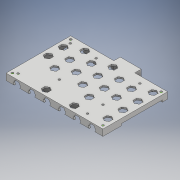
# Autodesk Inventor part: Housing Bottom
Saved by Autodesk Inventor 2017 (Build 210142000, 142)
## iProperties
Created: 2017-05-04
Part Number: Housing Bottom
Material: Generic
Document SubType Name: Modeling
Designer: andrew
Density: 1 g/cm^3
Appearance: Default
Author: andrew
Autodesk Inventor part; units mm, degrees
(part 1 of 3)
ref_plane "YZ Plane" through (0, 0, 0) normal (1, 0, 0) x (0, 1, 0)
ref_plane "XZ Plane" through (0, 0, 0) normal (0, 1, 0) x (-1, 0, 0)
ref_plane "XY Plane" through (0, 0, 0) normal (0, 0, 1) x (1, 0, 0)
sketch "Sketch1" plane through (0, 0, 0) normal (0, 0, 1) x (1, 0, 0)
  line L0 (0, 0) -> (122, 0) construction
  line L1 (122, 78) -> (0, 78) construction
  line L2 (0, 78) -> (0, 0) construction
  line L3 (122, 78) -> (124, 78) construction
  line L4 (124, 78) -> (124, 0) construction
  line L5 (124, 0) -> (122, 0) construction
  line L6 (122, 0) -> (122, 78) construction
  line L7 (0, 78) -> (124, 78) construction
  line L8 (124, 81) -> (0, 81) construction
  line L9 (0, 81) -> (0, 78) construction
  line L10 (124, 78) -> (124, 81) construction
  line L11 (124, 78) -> (124, 81) construction
  line L12 (0, 77.4184) -> (0, 81) construction
  line L13 (0, 81) -> (124, 81) construction
  line L14 (0, 81) -> (124, 81) construction
  line L15 (124, 0) -> (0, 0) construction
  line L16 (0, 0) -> (0, 81) construction
  line L17 (0, 81) -> (124, 81) construction
  line L18 (124, 81) -> (124, 0) construction
  line L19 (124, 0) -> (0, 0) construction
  line L20 (0, 0) -> (0, 81) construction
  line L21 (122, 78) -> (37, 78) construction
  line L22 (37, 78) -> (37, 22) construction
  line L23 (37, 22) -> (122, 22) construction
  line L24 (122, 22) -> (122, 78) construction
  line L25 (37, 22) -> (40.5, 22) construction
  line L26 (40.5, 22) -> (40.5, 25.5) construction
  line L27 (40.5, 25.5) -> (37, 25.5) construction
  line L28 (37, 25.5) -> (37, 22) construction
  line L29 (40.5, 25.5) -> (40.5, 74.5) construction
  circle A0 centre (40.5, 74.5) radius 1.375
  circle A1 centre (40.5, 25.5) radius 1.375
  circle A2 centre (98.5, 74.5) radius 1.375
  line L30 (0, 81) -> (124, 81) construction
  line L31 (124, 81) -> (124, 0) construction
  line L32 (124, 0) -> (0, 0) construction
  line L33 (0, 0) -> (0, 81) construction
  line L34 (124, 81.5) -> (0, 81.5) construction
  line L35 (122, -0.5) -> (-0.5, -0.5) construction
  line L36 (-0.5, -0.5) -> (-0.5, 78) construction
  line L37 (-0.5, 78) -> (-0.5, 81) construction
  line L38 (124, 81.5) -> (124.5, 81.5) construction
  line L39 (37, 78) -> (69, 78) construction
  line L40 (69, 78) -> (81, 78) construction
  line L41 (81, 78) -> (81, 90) construction
  line L42 (81, 90) -> (57, 90) construction
  line L43 (57, 90) -> (57, 78) construction
  line L44 (37, 78) -> (47.6, 78) construction
  line L45 (47.6, 78) -> (47.6, 82.811) construction
  line L46 (47.6, 82.811) -> (53.1, 82.811) construction
  line L47 (53.1, 82.811) -> (42.1, 82.811) construction
  line L48 (42.1, 82.811) -> (42.1, 78) construction
  line L49 (53.1, 82.811) -> (53.1, 78) construction
  line L50 (-0.5, -0.5) -> (124.5, -0.5) construction
  line L51 (124.5, -0.5) -> (124.5, 81.5) construction
  line L52 (124.5, 81.5) -> (-0.5, 81.5) construction
  line L53 (-0.5, 81.5) -> (-0.5, -0.5) construction
  line L54 (124.5, 81.5) -> (-0.5, 81.5) construction
  line L55 (-0.5, 81.5) -> (-0.5, -0.5) construction
  line L56 (-0.5, -0.5) -> (124.5, -0.5) construction
  line L57 (124.5, -0.5) -> (124.5, 81.5) construction
  line L58 (126.5, 83.5) -> (126.5, -2.5)
  line L59 (126.5, -2.5) -> (-2.5, -2.5)
  line L60 (-2.5, -2.5) -> (-2.5, 83.5)
  line L61 (40.5, 25.5) -> (98.5, 25.5) construction
  line L62 (98.5, 25.5) -> (98.5, 74.5) construction
  circle A3 centre (98.5, 25.5) radius 1.375
  line L63 (98.5, 74.5) -> (98.5, 5) construction
  line L64 (98.5, 74.5) -> (168, 74.5) construction
  line L65 (98.5, 5) -> (6.05, 5) construction
  line L66 (6.05, 5) -> (6.05, 74.5) construction
  circle A4 centre (6.05, 74.5) radius 1.375
  circle A5 centre (6.05, 5) radius 1.375
  line L67 (6.05, 73.125) -> (6.05, 72.125) construction
  line L68 (6.05, 72.125) -> (6.05, 69.1979) construction
  line L69 (6.05, 72.125) -> (-13.4592, 72.125) construction
  line L70 (6.05, 72.125) -> (6.05, 51.125) construction
  line L71 (6.05, 51.125) -> (-23.4653, 51.125) construction
  line L72 (-23.4653, 51.125) -> (-15.502, 54.0974) construction
  line L73 (-15.502, 54.0974) -> (-18.8258, 56.9365) construction
  line L74 (-18.8258, 56.9365) -> (-13.0091, 61.0912) construction
  line L75 (-13.0091, 61.0912) -> (-16.1944, 66.6309) construction
  line L76 (-16.1944, 66.6309) -> (-13.4592, 72.125) construction
  line L77 (6.05, 6.375) -> (6.05, 22.1104) construction
  line L78 (-2.5, 14.2427) -> (-2.5, 16.7927) construction
  line L79 (-2.5, 16.7927) -> (-2.5, 11.6927) construction
  line L80 (-2.5, 11.6927) -> (85.5, 11.6927) construction
  line L81 (85.5, 11.6927) -> (85.5, 16.7927) construction
  line L82 (85.5, 16.7927) -> (-2.5, 16.7927) construction
  circle A6 centre (98.5, 5) radius 1.375
  line L83 (83, 90) -> (83, 83.5) construction
  line L84 (83, 90) -> (83, 92) construction
  line L85 (55, 92) -> (55, 83.5) construction
  line L86 (-2.5, 83.5) -> (55, 83.5)
  line L87 (83, 83.5) -> (126.5, 83.5)
  line L88 (83, 92) -> (81, 92) construction
  line L89 (57, 92) -> (55, 92) construction
  line L90 (81, 92) -> (57, 92) construction
  line L91 (83, 83.5) -> (83, 92)
  line L92 (83, 92) -> (55, 92)
  line L93 (55, 92) -> (55, 83.5)
  dimension "d55" = 2.75
  dimension "d1" = 78
  dimension "d3" = 3
  dimension "d7" = 85
  dimension "d8" = 56
  dimension "d9" = 3.5
  dimension "d10" = 3.5
  dimension "d11" = 49
  dimension "d12" = 2.75
  dimension "d13" = 2.75
  dimension "d14" = 2.75
  dimension "d21" = 0.5
  dimension "d22" = 0.5
  dimension "d23" = 0.5
  dimension "d24" = 32
  dimension "d25" = 12
  dimension "d28" = 24
  dimension "d29" = 10.6
  dimension "d30" = 5.5
  dimension "d31" = 11
  dimension "d45" = 58
  dimension "d46" = 49
  dimension "d47" = 2.75
  dimension "d48" = 69.5
  dimension "d49" = 90
  dimension "d50" = 92.45
  dimension "d51" = 90
  dimension "d52" = 69.5
  dimension "d53" = 90
  dimension "d56" = 1
  dimension "d57" = 21
  dimension "d64" = 5.1
  dimension "d65" = 88
  dimension "d66" = 90
  dimension "d163" = 2.75
  dimension "d172" = 28
  constraints: 188 end point, 28 perpendicular, 22 parallel, 19 point on line, 15 horizontal, 5 centre point, 5 coincident, 4 collinear, 4 vertical, 2 vertical alignment, 8 other
  measures "d1" distance of L1.start L0.end
  measures "d3" distance of L8.start L7.end
  measures "d7" distance of L23.end L22.end
  measures "d8" distance of L22.end L21.end
  measures "d9" distance of L27.end L26.end
  measures "d10" distance of L26.end L25.end
  measures "d11" distance of L26.end L29.end
  measures "d12" diameter of A0
  measures "d13" diameter of A1
  measures "d14" diameter of A2
  measures "d21" distance between parallel lines of L8 L34
  measures "d22" distance between parallel lines of L2 L36
  measures "d23" distance of L34.start L38.end
  measures "d24" distance of L21.end L39.end
  measures "d25" distance of L39.end L40.end
  measures "d28" distance of L41.end L42.end
  measures "d29" distance of L21.end L44.end
  measures "d30" distance of L45.end L46.end
  measures "d31" distance of L46.end L47.end
  measures "d45" distance of L61.start L61.end
  measures "d46" distance of L61.end L62.end
  measures "d47" diameter of A3
  measures "d48" distance of L62.end L63.end
  measures "d49" angle of L63 L64
  measures "d50" distance of L63.end L65.end
  measures "d51" angle of L63 L65
  measures "d52" distance of L65.end L66.end
  measures "d53" angle of L65 L66
  measures "d56" distance of L67.start L67.end
  measures "d57" distance of L67.end L70.end
  measures "d64" distance of L78.end L79.end
  measures "d65" distance of L79.end L80.end
  measures "d66" angle of L80 L79
  measures "d163" diameter of A6
  measures "d172" distance of L84.end L85.start
extrude "Extrusion1" add sketch "Sketch1" along normal blind 2
sketch "Sketch2" plane through (0, 0, 0) normal (0, 0, -1) x (-1, 0, 0)
  circle A0 centre (-40.5, 74.5) radius 1.375 projected
  circle A1 centre (-40.5, 25.5) radius 1.375 projected
  circle A2 centre (-98.5, 74.5) radius 1.375 projected
  circle A3 centre (-98.5, 25.5) radius 1.375 projected
  circle A4 centre (-40.5, 74.5) radius 3
  circle A5 centre (-40.5, 25.5) radius 3
  circle A6 centre (-98.5, 74.5) radius 3
  circle A7 centre (-98.5, 25.5) radius 3
  line L0 (-126.5, 83.5) -> (-126.5, -2.5)
  circle A8 centre (-6.05, 74.5) radius 1.375
  line L1 (-6.05, 72.125) -> (-6.05, 69.1979) construction
  line L2 (-6.05, 72.125) -> (-6.05, 51.125) construction
  line L3 (-6.05, 72.125) -> (13.4592, 72.125) construction
  line L4 (16.1944, 66.6309) -> (13.4592, 72.125) construction
  line L5 (13.0091, 61.0912) -> (16.1944, 66.6309) construction
  line L6 (15.502, 54.0974) -> (18.8258, 56.9365) construction
  line L7 (-6.05, 51.125) -> (23.4653, 51.125) construction
  line L8 (23.4653, 51.125) -> (15.502, 54.0974) construction
  line L9 (18.8258, 56.9365) -> (13.0091, 61.0912) construction
  circle A9 centre (-6.05, 5) radius 1.375
  line L10 (-122, 78) -> (-37, 78) construction
  line L11 (-124, 81) -> (0, 81) construction
  line L12 (0, 81) -> (-124, 81) construction
  line L13 (0, 81) -> (-124, 81) construction
  line L14 (0, 81) -> (-124, 81) construction
  line L15 (0, 81) -> (-124, 81) construction
  line L16 (-124, 81.5) -> (0, 81.5) construction
  line L17 (-124.5, 81.5) -> (0.5, 81.5) construction
  line L18 (2.5, 83.5) -> (-126.5, 83.5)
  line L19 (-124.5, 81.5) -> (0.5, 81.5) construction
  line L20 (0, 78) -> (-124, 78) construction
  line L21 (0, 0) -> (-122, 0) construction
  line L22 (-122, 78) -> (0, 78) construction
  line L23 (-37, 78) -> (-69, 78) construction
  line L24 (-40.5, 25.5) -> (-40.5, 74.5) construction
  circle A10 centre (-40.5, 74.5) radius 1.375
  line L25 (0, 78) -> (0, 0) construction
  line L26 (-40.5, 25.5) -> (-37, 25.5) construction
  line L27 (-40.5, 22) -> (-40.5, 25.5) construction
  line L28 (-37, 22) -> (-40.5, 22) construction
  line L29 (0, 81) -> (0, 78) construction
  line L30 (0, 0) -> (0, 81) construction
  line L31 (0, 77.4184) -> (0, 81) construction
  line L32 (0, 0) -> (0, 81) construction
  line L33 (-37, 25.5) -> (-37, 22) construction
  line L34 (-37, 78) -> (-37, 22) construction
  line L35 (0.5, -0.5) -> (0.5, 78) construction
  line L36 (0.5, 81.5) -> (0.5, -0.5) construction
  line L37 (0.5, 81.5) -> (0.5, -0.5) construction
  line L38 (-85.5, 11.6927) -> (-85.5, 16.7927) construction
  line L39 (-37, 78) -> (-47.6, 78) construction
  line L40 (-47.6, 78) -> (-47.6, 82.811) construction
  line L41 (0.5, 78) -> (0.5, 81) construction
  line L42 (-6.05, 73.125) -> (-6.05, 72.125) construction
  line L43 (-42.1, 82.811) -> (-42.1, 78) construction
  line L44 (-47.6, 82.811) -> (-53.1, 82.811) construction
  line L45 (-53.1, 82.811) -> (-42.1, 82.811) construction
  line L46 (-6.05, 6.375) -> (-6.05, 22.1104) construction
  line L47 (2.5, 14.2427) -> (2.5, 16.7927) construction
  line L48 (2.5, 16.7927) -> (2.5, 11.6927) construction
  line L49 (-6.05, 5) -> (-6.05, 74.5) construction
  line L50 (0, 0) -> (0, 81) construction
  line L51 (2.5, -2.5) -> (2.5, 83.5)
  circle A11 centre (-98.5, 74.5) radius 1.375
  line L52 (-40.5, 25.5) -> (-98.5, 25.5) construction
  circle A12 centre (-40.5, 25.5) radius 1.375
  line L53 (-37, 22) -> (-122, 22) construction
  line L54 (-85.5, 16.7927) -> (2.5, 16.7927) construction
  line L55 (2.5, 11.6927) -> (-85.5, 11.6927) construction
  line L56 (-98.5, 5) -> (-6.05, 5) construction
  line L57 (-126.5, -2.5) -> (2.5, -2.5)
  line L58 (0.5, -0.5) -> (-124.5, -0.5) construction
  line L59 (0.5, -0.5) -> (-124.5, -0.5) construction
  line L60 (-124, 0) -> (0, 0) construction
  line L61 (-124, 0) -> (0, 0) construction
  line L62 (-124, 0) -> (0, 0) construction
  line L63 (-122, -0.5) -> (0.5, -0.5) construction
  line L64 (-122, 22) -> (-122, 78) construction
  line L65 (-124, 81) -> (-124, 0) construction
  line L66 (-124.5, -0.5) -> (-124.5, 81.5) construction
  line L67 (-124, 0) -> (-122, 0) construction
  line L68 (-122, 78) -> (-124, 78) construction
  line L69 (-124, 78) -> (-124, 81) construction
  line L70 (-124, 78) -> (-124, 81) construction
  line L71 (-124, 81) -> (-124, 0) construction
  line L72 (-124, 78) -> (-124, 0) construction
  line L73 (-122, 0) -> (-122, 78) construction
  circle A13 centre (-98.5, 25.5) radius 1.375
  line L74 (-98.5, 25.5) -> (-98.5, 74.5) construction
  line L75 (-98.5, 74.5) -> (-98.5, 5) construction
  line L76 (-124.5, -0.5) -> (-124.5, 81.5) construction
  line L77 (-124, 81.5) -> (-124.5, 81.5) construction
  line L78 (-69, 78) -> (-81, 78) construction
  line L79 (-81, 78) -> (-81, 90) construction
  line L80 (-81, 90) -> (-57, 90) construction
  line L81 (-57, 90) -> (-57, 78) construction
  line L82 (-53.1, 82.811) -> (-53.1, 78) construction
  circle A14 centre (-98.5, 5) radius 1.375
  circle A15 centre (-6.05, 74.5) radius 3
  circle A16 centre (-6.05, 5) radius 3
  circle A17 centre (-98.5, 5) radius 3
  point P0 (0, 0)
  point P1 (2.5, -2.5)
  dimension "d67" = 6
  dimension "d68" = 6
  dimension "d69" = 6
  dimension "d70" = 6
  dimension "d111" = 2.75
  dimension "d112" = 6
  dimension "d113" = 6
  dimension "d114" = 6
  dimension "d1062" = 92.45
  constraints: 166 end point, 17 point on line, 12 centre point, 12 coincident, 2 vertical alignment, 4 other
  measures "d67" diameter of A4
  measures "d68" diameter of A5
  measures "d69" diameter of A6
  measures "d70" diameter of A7
  measures "d111" diameter of A14
  measures "d112" diameter of A15
  measures "d113" diameter of A16
  measures "d114" diameter of A17
  measures "d1062" distance of L56.start L56.end
extrude "Extrusion2" add sketch "Sketch2" along normal blind 3 contours A4 | A5 | A6 | A7 | A15 | A16 | A17
draft "FaceDraft1" angle 15 pull direction (0, 0, -1) faces at (37.5097, 74.7414, -1) (37.5097, 25.2586, -2) (98.3792, 22.5024, -2) fixed edges at (43.5, 74.5, -3) (43.5, 25.5, -3) (101.5, 25.5, -3)
draft "FaceDraft2" angle 15 pull direction (0, 0, -1) faces at (98.3792, 71.5024, -2) (3.0597, 4.7586, -2) (95.5097, 4.7586, -2) (3.0597, 74.2586, -2) fixed edges at (101.5, 74.5, -3) (9.05, 5, -3) (101.5, 5, -3) (9.05, 74.5, -3)
sketch "Sketch3" plane through (0, 0, 0) normal (0, 0, -1) x (-1, 0, 0)
  circle A0 centre (-40.5, 74.5) radius 1.375
  line L0 (-42.1, 82.811) -> (-42.1, 78) construction
  line L1 (-40.5, 25.5) -> (-98.5, 25.5) construction
  line L2 (-40.5, 25.5) -> (-40.5, 74.5) construction
  line L3 (-122, 22) -> (-122, 78) construction
  line L4 (-40.5, 22) -> (-40.5, 25.5) construction
  line L5 (-37, 25.5) -> (-37, 22) construction
  line L6 (-37, 78) -> (-37, 22) construction
  line L7 (-37, 22) -> (-40.5, 22) construction
  line L8 (-37, 22) -> (-122, 22) construction
  line L9 (-124.5, -0.5) -> (-124.5, 81.5) construction
  line L10 (-124, 81) -> (-124, 0) construction
  circle A1 centre (-98.5, 25.5) radius 1.375
  line L11 (-124.5, -0.5) -> (-124.5, 81.5) construction
  line L12 (-126.5, 83.5) -> (-126.5, -2.5)
  line L13 (-98.5, 74.5) -> (-98.5, 5) construction
  line L14 (0, 0) -> (-122, 0) construction
  line L15 (-122, 0) -> (-122, 78) construction
  line L16 (-124, 78) -> (-124, 0) construction
  line L17 (-124, 81) -> (-124, 0) construction
  line L18 (-122, 78) -> (-124, 78) construction
  line L19 (-124, 78) -> (-124, 81) construction
  line L20 (-124, 78) -> (-124, 81) construction
  line L21 (-122, 78) -> (0, 78) construction
  line L22 (0, 78) -> (-124, 78) construction
  line L23 (-124, 81) -> (0, 81) construction
  line L24 (0, 81) -> (-124, 81) construction
  line L25 (0, 81) -> (-124, 81) construction
  line L26 (0, 81) -> (-124, 81) construction
  line L27 (-124, 81.5) -> (0, 81.5) construction
  line L28 (-124.5, 81.5) -> (0.5, 81.5) construction
  line L29 (-124.5, 81.5) -> (0.5, 81.5) construction
  line L30 (2.5, 83.5) -> (-126.5, 83.5)
  line L31 (0, 81) -> (-124, 81) construction
  line L32 (-40.5, 25.5) -> (-37, 25.5) construction
  circle A2 centre (-40.5, 25.5) radius 1.375
  line L33 (-98.5, 5) -> (-4.8, 5) construction
  line L34 (-124, 0) -> (-122, 0) construction
  line L35 (-124, 0) -> (0, 0) construction
  line L36 (-124, 0) -> (0, 0) construction
  line L37 (-124, 0) -> (0, 0) construction
  line L38 (-122, -0.5) -> (0.5, -0.5) construction
  line L39 (0.5, -0.5) -> (-124.5, -0.5) construction
  line L40 (0.5, -0.5) -> (-124.5, -0.5) construction
  line L41 (-126.5, -2.5) -> (2.5, -2.5)
  line L42 (0, 81) -> (0, 78) construction
  line L43 (0, 77.4184) -> (0, 81) construction
  line L44 (0, 0) -> (0, 81) construction
  line L45 (0, 0) -> (0, 81) construction
  line L46 (0.5, 78) -> (0.5, 81) construction
  line L47 (0.5, -0.5) -> (0.5, 78) construction
  line L48 (0, 0) -> (0, 81) construction
  line L49 (-4.8, 6.375) -> (-4.8, 22.1104) construction
  circle A3 centre (-4.8, 5) radius 1.375 construction
  line L50 (2.5, 14.2427) -> (2.5, 16.7927) construction
  line L51 (2.5, 16.7927) -> (2.5, 11.6927) construction
  line L52 (-4.8, 5) -> (-4.8, 74.5) construction
  line L53 (0.5, 81.5) -> (0.5, -0.5) construction
  line L54 (0.5, 81.5) -> (0.5, -0.5) construction
  line L55 (2.5, -2.5) -> (2.5, 83.5)
  line L56 (0, 78) -> (0, 0) construction
  line L57 (-98.5, 25.5) -> (-98.5, 74.5) construction
  line L58 (-98.5, 74.5) -> (-168, 74.5) construction
  circle A4 centre (-98.5, 74.5) radius 1.375
  circle A5 centre (-4.8, 74.5) radius 1.375 construction
  line L59 (-4.8, 72.125) -> (-4.8, 69.1979) construction
  line L60 (-4.8, 72.125) -> (-4.8, 51.125) construction
  line L61 (-4.8, 73.125) -> (-4.8, 72.125) construction
  line L62 (-4.8, 72.125) -> (14.7092, 72.125) construction
  line L63 (14.2591, 61.0912) -> (17.4444, 66.6309) construction
  line L64 (16.752, 54.0974) -> (20.0758, 56.9365) construction
  line L65 (20.0758, 56.9365) -> (14.2591, 61.0912) construction
  line L66 (-4.8, 51.125) -> (24.7153, 51.125) construction
  line L67 (24.7153, 51.125) -> (16.752, 54.0974) construction
  line L68 (17.4444, 66.6309) -> (14.7092, 72.125) construction
  line L69 (-53.1, 82.811) -> (-42.1, 82.811) construction
  line L70 (-37, 78) -> (-47.6, 78) construction
  line L71 (-47.6, 78) -> (-47.6, 82.811) construction
  line L72 (-47.6, 82.811) -> (-53.1, 82.811) construction
  line L73 (-53.1, 82.811) -> (-53.1, 78) construction
  line L74 (-81, 78) -> (-81, 90) construction
  line L75 (-81, 90) -> (-57, 90) construction
  line L76 (-57, 90) -> (-57, 78) construction
  line L77 (-69, 78) -> (-81, 78) construction
  line L78 (-124, 81.5) -> (-124.5, 81.5) construction
  line L79 (-37, 78) -> (-69, 78) construction
  line L80 (-122, 78) -> (-37, 78) construction
  line L81 (2.5, 16.7927) -> (2.5, 17.7927)
  line L82 (2.5, 83.5) -> (2.5, -2.5) projected
  line L83 (2.5, 17.7927) -> (-87.0105, 17.7927)
  line L84 (2.5, 11.6927) -> (2.5, 10.6927)
  line L85 (2.5, 10.6927) -> (-87.0105, 10.6927)
  line L86 (-87.0105, 10.6927) -> (-87.0105, 17.7927)
  line L87 (-83, 83.5) -> (-83, 92) construction
  line L88 (-83, 92) -> (-55, 92) construction
  line L89 (-55, 92) -> (-55, 83.5) construction
  point P0 (0, 0)
  dimension "d155" = 1
  dimension "d156" = 1
  constraints: 172 end point, 19 point on line, 4 centre point, 4 coincident, 3 perpendicular, 2 vertical alignment, 4 other
  measures "d155" distance of L50.end L81.end
  measures "d156" distance of L51.end L84.end
extrude "Extrusion3" add sketch "Sketch3" along normal blind 6 contours L55 L85 L86 L83
sketch "Sketch4" plane through (-2.5, -2.5, 2) normal (-1, 0, 0) x (0, 0, 1)
  line L0 (-5, 16.7427) -> (-5, 19.4927) construction
  circle A0 centre (-5, 16.7427) radius 2.75
  point P0 (-2, 2.5)
  dimension "d154" = 5.5
  constraints: 2 end point, 1 centre point, 1 coincident
  measures "d154" diameter of A0
extrude "Extrusion4" cut sketch "Sketch4" against normal blind 88
sketch "Sketch5" plane through (-2.5, -2.5, 2) normal (-1, 0, 0) x (0, 0, 1)
  circle A0 centre (-5, 16.7427) radius 2.75 projected
  line L0 (-5, 16.7427) -> (-5, 19.4927)
  line L1 (-5, 16.7427) -> (-5, 13.9927)
  line L2 (-5, 13.9927) -> (-10.5989, 13.9927)
  line L3 (-10.5989, 13.9927) -> (-10.5989, 19.4927)
  line L4 (-10.5989, 19.4927) -> (-5, 19.4927)
  point P0 (-2, 2.5)
  constraints: 10 end point, 2 perpendicular, 2 point on circle, 1 horizontal, 1 point on line, 1 tangent
extrude "Extrusion5" cut sketch "Sketch5" against normal blind 14 contours L0 L1 A0 | A0 L2 L3 L4 picked at (-5.2194, 14.936)
sketch "Sketch8" plane through (0, 0, 0) normal (0, 0, -1) x (-1, 0, 0)
  line L0 (2.5, 10.6927) -> (-87.0105, 10.6927) projected
  line L1 (-87.0105, 10.6927) -> (-87.0105, 17.7927) projected
  line L2 (-87.0105, 17.7927) -> (2.5, 17.7927) projected
  line L3 (2.5, 83.5) -> (2.5, 17.7927) projected
  line L4 (-55, 83.5) -> (2.5, 83.5) projected
  line L5 (-55, 92) -> (-55, 83.5) projected
  line L6 (-83, 92) -> (-55, 92) projected
  line L7 (-83, 83.5) -> (-83, 92) projected
  line L8 (-126.5, 83.5) -> (-83, 83.5) projected
  line L9 (-126.5, -2.5) -> (-126.5, 83.5) projected
  line L10 (2.5, -2.5) -> (-126.5, -2.5) projected
  line L11 (2.5, 10.6927) -> (2.5, -2.5) projected
  circle A0 centre (-6.05, 5) radius 3.8038 projected
  circle A1 centre (-98.5, 25.5) radius 3.8038 projected
  circle A2 centre (-40.5, 25.5) radius 3.8038 projected
  circle A3 centre (-40.5, 74.5) radius 3.8038 projected
  circle A4 centre (-98.5, 74.5) radius 3.8038 projected
  circle A5 centre (-6.05, 74.5) radius 3.8038 projected
  circle A6 centre (-98.5, 5) radius 3.8038 projected
  line L12 (-124.5, 81.5) -> (-81, 81.5)
  line L13 (-81, 81.5) -> (-81, 90)
  line L14 (-81, 90) -> (-57, 90)
  line L15 (-57, 90) -> (-57, 81.5)
  line L16 (-57, 81.5) -> (0.5, 81.5)
  line L17 (0.5, 81.5) -> (0.5, 17.7927)
  line L18 (0.5, 10.6927) -> (0.5, -0.5)
  line L19 (0.5, -0.5) -> (-124.5, -0.5)
  line L20 (-124.5, -0.5) -> (-124.5, 81.5)
  line L21 (0.5, 17.7927) -> (2.5, 17.7927)
  line L22 (0.5, 10.6927) -> (2.5, 10.6927)
  point P0 (0, 0)
  dimension "d180" = 2
  constraints: 22 end point, 2 point on line, 1 collinear, 1 horizontal, 5 other
  measures "d180" distance between parallel lines of L9 L20
extrude "Extrusion7" add sketch "Sketch8" along normal blind 4.25 contours L11 L10 L9 L8 L7 L6 L5 L4 L3 L2 L17 L16 L15 L14 L13 L12 L20 L19 L18 L0
sketch "Sketch9" plane through (0, 0, -4.25) normal (0, 0, -1) x (-1, 0, 0)
  line L0 (-4.8, 72.125) -> (14.7092, 72.125) construction
  line L1 (14.2591, 61.0912) -> (17.4444, 66.6309) construction
  line L2 (17.4444, 66.6309) -> (14.7092, 72.125) construction
  line L3 (16.752, 54.0974) -> (20.0758, 56.9365) construction
  line L4 (20.0758, 56.9365) -> (14.2591, 61.0912) construction
  line L5 (-4.8, 51.125) -> (24.7153, 51.125) construction
  line L6 (24.7153, 51.125) -> (16.752, 54.0974) construction
  line L7 (-37, 78) -> (-37, 22) construction
  line L8 (-40.5, 22) -> (-40.5, 25.5) construction
  line L9 (-40.5, 25.5) -> (-37, 25.5) construction
  line L10 (-40.5, 25.5) -> (-40.5, 74.5) construction
  circle A0 centre (-40.5, 25.5) radius 1.375 construction
  circle A1 centre (-40.5, 74.5) radius 1.375 construction
  line L11 (-37, 25.5) -> (-37, 22) construction
  line L12 (-37, 22) -> (-40.5, 22) construction
  circle A2 centre (-4.8, 5) radius 1.375 construction
  line L13 (2.5, 14.2427) -> (2.5, 16.7927) construction
  line L14 (2.5, 16.7927) -> (2.5, 11.6927) construction
  line L15 (-98.5, 5) -> (-4.8, 5) construction
  line L16 (0, 0) -> (-122, 0) construction
  line L17 (-122, -0.5) -> (0.5, -0.5) construction
  line L18 (-126.5, -2.5) -> (2.5, -2.5) construction
  line L19 (0.5, -0.5) -> (-124.5, -0.5) construction
  line L20 (0.5, -0.5) -> (-124.5, -0.5) construction
  line L21 (-124, 0) -> (0, 0) construction
  line L22 (-124, 0) -> (0, 0) construction
  line L23 (-124, 0) -> (0, 0) construction
  line L24 (-37, 22) -> (-122, 22) construction
  line L25 (-40.5, 25.5) -> (-98.5, 25.5) construction
  line L26 (-98.5, 25.5) -> (-98.5, 74.5) construction
  line L27 (-122, 22) -> (-122, 78) construction
  line L28 (-98.5, 74.5) -> (-98.5, 5) construction
  line L29 (-124, 81) -> (-124, 0) construction
  line L30 (-124, 81) -> (-124, 0) construction
  line L31 (-122, 0) -> (-122, 78) construction
  line L32 (-124, 78) -> (-124, 0) construction
  circle A3 centre (-98.5, 25.5) radius 1.375 construction
  line L33 (-124, 0) -> (-122, 0) construction
  circle A4 centre (-98.5, 74.5) radius 1.375 construction
  line L34 (-124, 81.5) -> (-124.5, 81.5) construction
  line L35 (-98.5, 74.5) -> (-168, 74.5) construction
  line L36 (-4.8, 6.375) -> (-4.8, 22.1104) construction
  line L37 (-42.1, 82.811) -> (-42.1, 78) construction
  line L38 (-122, 78) -> (-124, 78) construction
  line L39 (-124, 78) -> (-124, 81) construction
  line L40 (-122, 78) -> (0, 78) construction
  line L41 (0, 78) -> (-124, 78) construction
  line L42 (2.5, 83.5) -> (-126.5, 83.5) construction
  line L43 (-124.5, 81.5) -> (0.5, 81.5) construction
  line L44 (-124.5, 81.5) -> (0.5, 81.5) construction
  line L45 (-124, 78) -> (-124, 81) construction
  line L46 (-124, 81) -> (0, 81) construction
  line L47 (0, 81) -> (-124, 81) construction
  line L48 (0, 81) -> (-124, 81) construction
  line L49 (0, 81) -> (-124, 81) construction
  line L50 (-124, 81.5) -> (0, 81.5) construction
  line L51 (0, 81) -> (-124, 81) construction
  line L52 (-4.8, 5) -> (-4.8, 74.5) construction
  line L53 (0, 78) -> (0, 0) construction
  line L54 (0.5, -0.5) -> (0.5, 78) construction
  line L55 (0, 0) -> (0, 81) construction
  line L56 (0, 0) -> (0, 81) construction
  line L57 (0, 0) -> (0, 81) construction
  line L58 (0.5, 81.5) -> (0.5, -0.5) construction
  line L59 (0.5, 81.5) -> (0.5, -0.5) construction
  line L60 (2.5, -2.5) -> (2.5, 83.5) construction
  line L61 (-4.8, 72.125) -> (-4.8, 51.125) construction
  line L62 (-4.8, 72.125) -> (-4.8, 69.1979) construction
  line L63 (-4.8, 73.125) -> (-4.8, 72.125) construction
  circle A5 centre (-4.8, 74.5) radius 1.375 construction
  line L64 (0, 81) -> (0, 78) construction
  line L65 (0, 77.4184) -> (0, 81) construction
  line L66 (0.5, 78) -> (0.5, 81) construction
  line L67 (-81, 78) -> (-81, 90) construction
  line L68 (-69, 78) -> (-81, 78) construction
  line L69 (-122, 78) -> (-37, 78) construction
  line L70 (-57, 90) -> (-57, 78) construction
  line L71 (-53.1, 82.811) -> (-53.1, 78) construction
  line L72 (-47.6, 78) -> (-47.6, 82.811) construction
  line L73 (-47.6, 82.811) -> (-53.1, 82.811) construction
  line L74 (-53.1, 82.811) -> (-42.1, 82.811) construction
  line L75 (-37, 78) -> (-47.6, 78) construction
  line L76 (-37, 78) -> (-69, 78) construction
  line L77 (-81, 90) -> (-57, 90) construction
  line L78 (2.5, 16.7927) -> (2.5, 17.7927) construction
  line L79 (2.5, 83.5) -> (2.5, -2.5) construction
  line L80 (2.5, 17.7927) -> (-87.0105, 17.7927) construction
  line L81 (2.5, 11.6927) -> (2.5, 10.6927) construction
  line L82 (2.5, 10.6927) -> (-87.0105, 10.6927) construction
  line L83 (-87.0105, 10.6927) -> (-87.0105, 17.7927) construction
  line L84 (-83, 83.5) -> (-83, 92) construction
  line L85 (-83, 92) -> (-55, 92) construction
  line L86 (-55, 92) -> (-55, 83.5) construction
  line L87 (0.5, 81.5) -> (-57, 81.5) projected
  line L88 (-53.1, 81.5) -> (-53.1, 83.5)
  line L89 (-42.1, 81.5) -> (-42.1, 83.5)
  line L90 (-124.5, 81) -> (-126.5, 81)
  line L91 (-126.5, -2.5) -> (-126.5, 83.5) projected
  line L92 (0.5, 10.6927) -> (2.5, 10.6927) projected
  line L93 (0.5, 10.6927) -> (0.5, -0.5) projected
  line L94 (0.5, -0.5) -> (-124.5, -0.5) projected
  line L95 (-124.5, -0.5) -> (-124.5, 81.5) projected
  line L96 (-124.5, 81.5) -> (-81, 81.5) projected
  line L97 (-81, 81.5) -> (-81, 90) projected
  line L98 (-81, 90) -> (-57, 90) projected
  line L99 (-57, 90) -> (-57, 81.5) projected
  line L100 (-57, 81.5) -> (0.5, 81.5) projected
  line L101 (0.5, 81.5) -> (0.5, 17.7927) projected
  line L102 (2.5, 17.7927) -> (0.5, 17.7927) projected
  line L103 (2.5, 17.7927) -> (2.5, 83.5) projected
  line L104 (2.5, 83.5) -> (-55, 83.5) projected
  line L105 (-55, 83.5) -> (-55, 92) projected
  line L106 (-55, 92) -> (-83, 92) projected
  line L107 (-83, 92) -> (-83, 83.5) projected
  line L108 (-83, 83.5) -> (-126.5, 83.5) projected
  line L109 (-126.5, 83.5) -> (-126.5, -2.5) projected
  line L110 (-126.5, -2.5) -> (2.5, -2.5) projected
  line L111 (2.5, -2.5) -> (2.5, 10.6927) projected
  line L112 (-122, 22) -> (-124, 22)
  line L113 (-124.5, 22) -> (-126.5, 22)
  line L114 (-126.5, 83.5) -> (-126.5, 81) construction
  line L115 (-126.5, 22) -> (-126.5, -2.5) construction
  line L116 (-124.5, -0.5) -> (-124.5, 22) construction
  line L117 (-124.5, 81) -> (-124.5, 81.5) construction
  line L118 (-124.5, -0.5) -> (-124.5, 22) construction
  line L119 (-124.5, 81) -> (-124.5, 81.5) construction
  point P0 (0, 0)
  point P1 (0, 0)
  dimension "d183" = 1
  dimension "d184" = 1
  dimension "d185" = 11
  constraints: 196 end point, 32 point on line, 4 centre point, 4 coincident, 3 perpendicular, 2 parallel, 2 vertical alignment, 4 other
  measures "d183" distance of L13.end L80.start
  measures "d184" distance of L14.end L82.start
  measures "d185" distance between parallel lines of L37 L71
extrude "Extrusion8" add sketch "Sketch9" along normal blind 15.98
sketch "Sketch10" plane through (0, 0, -20.23) normal (0, 0, -1) x (-1, 0, 0)
  line L0 (-4.8, 72.125) -> (14.7092, 72.125) construction
  line L1 (-4.8, 51.125) -> (24.7153, 51.125) construction
  line L2 (17.4444, 66.6309) -> (14.7092, 72.125) construction
  line L3 (14.2591, 61.0912) -> (17.4444, 66.6309) construction
  line L4 (20.0758, 56.9365) -> (14.2591, 61.0912) construction
  line L5 (16.752, 54.0974) -> (20.0758, 56.9365) construction
  line L6 (24.7153, 51.125) -> (16.752, 54.0974) construction
  circle A0 centre (-4.8, 5) radius 1.375 construction
  line L7 (-126.5, -2.5) -> (2.5, -2.5) construction
  line L8 (0.5, -0.5) -> (-124.5, -0.5) construction
  line L9 (0.5, -0.5) -> (-124.5, -0.5) construction
  line L10 (-124, 0) -> (0, 0) construction
  line L11 (-124, 0) -> (0, 0) construction
  line L12 (-124, 0) -> (0, 0) construction
  line L13 (0, 0) -> (-122, 0) construction
  line L14 (-122, -0.5) -> (0.5, -0.5) construction
  line L15 (-98.5, 5) -> (-4.8, 5) construction
  line L16 (2.5, 17.7927) -> (-87.0105, 17.7927) construction
  line L17 (2.5, 14.2427) -> (2.5, 16.7927) construction
  line L18 (2.5, 16.7927) -> (2.5, 11.6927) construction
  line L19 (2.5, 10.6927) -> (-87.0105, 10.6927) construction
  line L20 (-37, 78) -> (-37, 22) construction
  line L21 (-40.5, 25.5) -> (-37, 25.5) construction
  line L22 (-40.5, 25.5) -> (-40.5, 74.5) construction
  circle A1 centre (-40.5, 74.5) radius 1.375 construction
  line L23 (-98.5, 25.5) -> (-98.5, 74.5) construction
  line L24 (-42.1, 82.811) -> (-42.1, 78) construction
  line L25 (-122, 78) -> (0, 78) construction
  line L26 (0, 78) -> (-124, 78) construction
  line L27 (2.5, 83.5) -> (-126.5, 83.5) construction
  line L28 (-124.5, 81.5) -> (0.5, 81.5) construction
  line L29 (-124.5, 81.5) -> (0.5, 81.5) construction
  line L30 (0, 81) -> (-124, 81) construction
  line L31 (0, 81) -> (-124, 81) construction
  line L32 (0, 81) -> (-124, 81) construction
  line L33 (-124, 81) -> (0, 81) construction
  line L34 (-124, 81.5) -> (0, 81.5) construction
  line L35 (0, 81) -> (-124, 81) construction
  line L36 (-40.5, 22) -> (-40.5, 25.5) construction
  circle A2 centre (-40.5, 25.5) radius 1.375 construction
  line L37 (-37, 25.5) -> (-37, 22) construction
  line L38 (-37, 22) -> (-40.5, 22) construction
  line L39 (-37, 22) -> (-122, 22) construction
  line L40 (-40.5, 25.5) -> (-98.5, 25.5) construction
  circle A3 centre (-98.5, 74.5) radius 1.375 construction
  line L41 (-122, 78) -> (-124, 78) construction
  line L42 (-122, 22) -> (-122, 78) construction
  line L43 (-98.5, 74.5) -> (-98.5, 5) construction
  line L44 (-124, 81) -> (-124, 0) construction
  line L45 (-124, 81) -> (-124, 0) construction
  line L46 (-122, 0) -> (-122, 78) construction
  line L47 (-124, 78) -> (-124, 0) construction
  line L48 (-124, 78) -> (-124, 81) construction
  line L49 (-124, 81.5) -> (-124.5, 81.5) construction
  line L50 (2.5, 16.7927) -> (2.5, 17.7927) construction
  line L51 (2.5, 11.6927) -> (2.5, 10.6927) construction
  line L52 (-4.8, 6.375) -> (-4.8, 22.1104) construction
  line L53 (-4.8, 5) -> (-4.8, 74.5) construction
  line L54 (0, 78) -> (0, 0) construction
  line L55 (0.5, -0.5) -> (0.5, 78) construction
  line L56 (2.5, -2.5) -> (2.5, 83.5) construction
  line L57 (2.5, 83.5) -> (2.5, -2.5) construction
  line L58 (0.5, 81.5) -> (0.5, -0.5) construction
  line L59 (0.5, 81.5) -> (0.5, -0.5) construction
  line L60 (0, 0) -> (0, 81) construction
  line L61 (0, 0) -> (0, 81) construction
  line L62 (0, 0) -> (0, 81) construction
  circle A4 centre (-98.5, 25.5) radius 1.375 construction
  line L63 (-124, 0) -> (-122, 0) construction
  line L64 (-87.0105, 10.6927) -> (-87.0105, 17.7927) construction
  line L65 (-98.5, 74.5) -> (-168, 74.5) construction
  line L66 (-124, 78) -> (-124, 81) construction
  line L67 (0, 81) -> (0, 78) construction
  line L68 (-4.8, 72.125) -> (-4.8, 51.125) construction
  line L69 (-4.8, 72.125) -> (-4.8, 69.1979) construction
  line L70 (-4.8, 73.125) -> (-4.8, 72.125) construction
  circle A5 centre (-4.8, 74.5) radius 1.375 construction
  line L71 (0, 77.4184) -> (0, 81) construction
  line L72 (0.5, 78) -> (0.5, 81) construction
  line L73 (-81, 78) -> (-81, 90) construction
  line L74 (-53.1, 82.811) -> (-53.1, 78) construction
  line L75 (-47.6, 78) -> (-47.6, 82.811) construction
  line L76 (-47.6, 82.811) -> (-53.1, 82.811) construction
  line L77 (-53.1, 82.811) -> (-42.1, 82.811) construction
  line L78 (-37, 78) -> (-47.6, 78) construction
  line L79 (-37, 78) -> (-69, 78) construction
  line L80 (-57, 90) -> (-57, 78) construction
  line L81 (-55, 92) -> (-55, 83.5) construction
  line L82 (-81, 90) -> (-57, 90) construction
  line L83 (-122, 78) -> (-37, 78) construction
  line L84 (-83, 92) -> (-55, 92) construction
  line L85 (-83, 83.5) -> (-83, 92) construction
  line L86 (-69, 78) -> (-81, 78) construction
  line L87 (0.5, 81.5) -> (-57, 81.5) construction
  line L88 (-53.1, 81.5) -> (-53.1, 83.5) construction
  line L89 (-42.1, 81.5) -> (-42.1, 83.5) construction
  line L90 (-126.5, -2.5) -> (-126.5, 83.5) construction
  line L91 (0.5, 10.6927) -> (2.5, 10.6927) construction
  line L92 (0.5, 10.6927) -> (0.5, -0.5) construction
  line L93 (0.5, -0.5) -> (-124.5, -0.5) construction
  line L94 (-124.5, -0.5) -> (-124.5, 81.5) construction
  line L95 (-124.5, 81.5) -> (-81, 81.5) construction
  line L96 (-81, 81.5) -> (-81, 90) construction
  line L97 (-81, 90) -> (-57, 90) construction
  line L98 (-57, 90) -> (-57, 81.5) construction
  line L99 (-57, 81.5) -> (0.5, 81.5) construction
  line L100 (0.5, 81.5) -> (0.5, 17.7927) construction
  line L101 (2.5, 17.7927) -> (0.5, 17.7927) construction
  line L102 (2.5, 17.7927) -> (2.5, 83.5) construction
  line L103 (2.5, 83.5) -> (-55, 83.5) construction
  line L104 (-55, 83.5) -> (-55, 92) construction
  line L105 (-55, 92) -> (-83, 92) construction
  line L106 (-83, 92) -> (-83, 83.5) construction
  line L107 (-83, 83.5) -> (-126.5, 83.5) construction
  line L108 (-126.5, -2.5) -> (2.5, -2.5) construction
  line L109 (2.5, -2.5) -> (2.5, 10.6927) construction
  line L110 (-122, 22) -> (-124, 22) construction
  line L111 (-124.5, 22) -> (-126.5, 22) construction
  line L112 (-126.5, 83.5) -> (-126.5, 81) construction
  line L113 (-126.5, 22) -> (-126.5, -2.5) construction
  line L114 (-124.5, -0.5) -> (-124.5, 22) construction
  line L115 (-124.5, 81) -> (-124.5, 81.5) construction
  line L116 (-124.5, -0.5) -> (-124.5, 22) construction
  line L117 (-124.5, 81) -> (-124.5, 81.5) construction
  line L118 (-126.5, 22) -> (-124.5, 22)
  line L119 (-124.5, 22) -> (-124.5, 76.5)
  line L120 (-124.5, 81) -> (-126.5, 81)
  line L121 (-126.5, 76.5) -> (-126.5, 22)
  line L122 (-42.1, 81.5) -> (-53.1, 81.5)
  line L123 (-53.1, 81.5) -> (-53.1, 83.5)
  line L124 (-53.1, 83.5) -> (-42.1, 83.5)
  line L125 (-42.1, 83.5) -> (-42.1, 81.5)
  line L126 (-126.5, 83.5) -> (-126.5, -2.5) projected
  line L127 (-126.5, 76.5) -> (-124.5, 76.5)
  line L128 (-124.5, 81.5) -> (-124.5, -0.5) projected
  line L129 (-126.5, 83.5) -> (-126.5, 81) construction
  line L130 (-126.5, 76.5) -> (-126.5, -2.5) construction
  point P0 (0, 0)
  point P1 (0, 0)
  point P2 (0, 0)
  dimension "d188" = 1
  dimension "d189" = 1
  dimension "d190" = 11
  constraints: 258 end point, 34 point on line, 6 perpendicular, 4 centre point, 4 coincident, 4 parallel, 2 horizontal, 2 vertical alignment, 4 other
  measures "d188" distance of L17.end L16.start
  measures "d189" distance of L18.end L19.start
  measures "d190" distance between parallel lines of L24 L74
extrude "Extrusion9" cut sketch "Sketch10" against normal blind 16.23 contours L121 L127 L119 L118 | L122 L123 L124 L125
sketch "Sketch11" plane through (-2.5, -2.5, 2) normal (-1, 0, 0) x (0, 0, 1)
  arc A0 (-5, 13.9927) -> (-5, 19.4927) centre (-5, 16.7427) ccw projected
  line L0 (-2.25, 16.7427) -> (-9.61, 16.7427)
  line L1 (-9.61, 16.7427) -> (-10.61, 16.7427)
  line L2 (-10.61, 16.7427) -> (-10.61, 19.4927)
  line L3 (-8, 20.2927) -> (-22.23, 20.2927) projected
  line L4 (-8, 13.1927) -> (-22.23, 13.1927) projected
  line L5 (-10.81, 20.2927) -> (-22.23, 20.2927)
  line L6 (-22.23, 20.2927) -> (-22.23, 13.1927)
  line L7 (-22.23, 13.1927) -> (-10.81, 13.1927)
  line L8 (-10.61, 13.9927) -> (-10.61, 19.4927)
  line L9 (-8, 13.1927) -> (-8, 13.9927) projected
  line L10 (-8, 13.9927) -> (-10.61, 13.9927)
  line L11 (-10.81, 13.1927) -> (-8, 13.1927)
  line L12 (-8, 13.1927) -> (-8, 13.9927)
  line L13 (-8, 19.4927) -> (-8, 20.2927) projected
  line L14 (-8, 19.4927) -> (-10.61, 19.4927)
  line L15 (-10.81, 20.2927) -> (-8, 20.2927)
  line L16 (-8, 20.2927) -> (-8, 19.4927)
  point P0 (-2, 2.5)
  dimension "d193" = 7.36
  dimension "d194" = 1
  constraints: 26 end point, 4 horizontal, 4 parallel, 2 perpendicular, 2 point on line, 1 point on circle
  measures "d193" distance of L0.start L0.end
  measures "d194" distance of L0.end L1.end
extrude "Extrusion10" add sketch "Sketch11" against normal blind 2
sketch "Sketch13" plane through (-2.5, -2.5, 2) normal (-1, 0, 0) x (0, 0, 1)
  line L0 (-8, 20.2927) -> (-2, 20.2927) construction
  line L1 (-2, 20.2927) -> (-8, 20.2927) construction
  line L2 (-8, 19.4927) -> (-8, 20.2927) construction
  line L3 (-8, 20.2927) -> (-8, 13.1927) construction
  line L4 (-8, 13.1927) -> (-8, 13.9927) construction
  line L5 (-8, 13.9927) -> (-8, 19.4927) construction
  line L6 (-4.4826, 20.7927) -> (-4.4826, 25.0927) construction
  line L7 (-3.7587, 25.0927) -> (-2.5174, 22.9427) construction
  line L8 (-2.5174, 22.9427) -> (-3.7587, 20.7927) construction
  line L9 (-3.2413, 20.7927) -> (-5.7239, 20.7927) construction
  line L10 (-6.2413, 20.7927) -> (-7.4826, 22.9427) construction
  line L11 (-7.4826, 22.9427) -> (-6.2413, 25.0927) construction
  line L12 (-6.2413, 25.0927) -> (-3.7587, 25.0927) construction
  arc A0 (-5, 19.4927) -> (-5, 13.9927) centre (-5, 16.7427) ccw construction
  line L13 (-5, 17.2427) -> (-5, 20.7927) construction
  line L14 (-5, 20.7927) -> (-5, 22.9427) construction
  circle A1 centre (-5, 22.9427) radius 1.5 construction
  line L15 (-5.7239, 25.0927) -> (-5.7239, 27.0927) construction
  line L16 (-5.7239, 27.0927) -> (-2, 27.125) construction
  line L17 (-2, 27.125) -> (-5.7239, 27.0927)
  line L18 (-5.7239, 25.0927) -> (-5.7239, 27.0927)
  line L19 (-5.7239, 25.0927) -> (-3.7587, 25.0927)
  line L20 (-3.7587, 25.0927) -> (-2.5174, 22.9427)
  line L21 (-2.5174, 22.9427) -> (-3.7587, 20.7927)
  line L22 (-3.7587, 20.7927) -> (-3.7587, 20.5732)
  line L23 (-3.7587, 20.5732) -> (-1.7194, 20.5732)
  line L24 (-1.7194, 20.5732) -> (-1.7194, 27.125)
  line L25 (-2, 27.125) -> (-1.7194, 27.125)
  line L26 (-9.2411, 28.6649) -> (-9.2411, 29.1649)
  point P0 (-2, 2.5)
  point P1 (-4.4826, 22.9427)
  dimension "d197" = 4.3
  dimension "d199" = 3
  dimension "d200" = 2
  dimension "d1050" = 0.5
  constraints: 42 end point, 4 vertical, 3 collinear, 1 centre point, 1 coincident, 1 horizontal, 1 midpoint, 1 perpendicular, 1 point on line, 1 other
  measures "d197" distance of L6.start L6.end
  measures "d199" diameter of A1
  measures "d200" distance of L15.start L15.end
  measures "d1050" distance of L26.start L26.end
extrude "Extrusion11" add sketch "Sketch13" against normal blind 4.6
sketch "Sketch14" plane through (2.1, -2.5, 2) normal (1, 0, 0) x (0, 0, -1)
  line L0 (0, 86) -> (0, 0) construction
  line L1 (3.7587, 20.7927) -> (2.5174, 22.9427) construction
  line L2 (2.5174, 22.9427) -> (3.7587, 25.0927) construction
  line L3 (3.7587, 25.0927) -> (5.7239, 25.0927) construction
  line L4 (5.7239, 25.0927) -> (5.7239, 27.0927) construction
  line L5 (5.7239, 27.0927) -> (2, 27.125) projected
  line L6 (2, 20.5732) -> (2, 27.125) construction
  line L7 (2, 27.0927) -> (2, 20.7927)
  line L8 (2, 20.7927) -> (5.7239, 20.7927)
  line L9 (5.7239, 20.7927) -> (5.7239, 27.0927)
  line L10 (2, 20.5732) -> (3.7587, 20.5732) projected
  line L11 (3.7587, 20.5732) -> (3.7587, 20.7927) projected
  line L12 (2, 27.125) -> (2, 27.0927)
  line L13 (2, 20.5732) -> (2, 27.125) projected
  point P0 (2, 2.5)
  constraints: 8 end point, 1 collinear, 1 parallel
extrude "Extrusion12" add sketch "Sketch14" along normal blind 2 contours L9 L8 L7 L12 L5
sketch "Sketch15" plane through (-2.5, -2.5, 2) normal (-1, 0, 0) x (0, 0, 1)
  line L0 (-8, 20.7927) -> (-2, 20.7927) construction
  line L1 (-2, 20.7927) -> (-8, 20.7927) construction
  line L2 (-8, 19.7927) -> (-8, 20.7927) construction
  line L3 (-8, 20.7927) -> (-8, 13.6927) construction
  line L4 (-8, 13.1927) -> (-8, 14.1927) construction
  line L5 (-8, 14.1927) -> (-8, 19.2927) construction
  line L6 (-4.4826, 20.7927) -> (-4.4826, 25.0927) construction
  line L7 (-3.7587, 25.0927) -> (-2.5174, 22.9427) construction
  line L8 (-2.5174, 22.9427) -> (-3.7587, 20.7927) construction
  line L9 (-3.2413, 20.7927) -> (-5.7239, 20.7927) construction
  line L10 (-6.2413, 20.7927) -> (-7.4826, 22.9427) construction
  line L11 (-7.4826, 22.9427) -> (-6.2413, 25.0927) construction
  line L12 (-6.2413, 25.0927) -> (-3.7587, 25.0927) construction
  arc A0 (-5, 19.2927) -> (-5, 14.1927) centre (-5, 16.7427) ccw construction
  line L13 (-5, 17.2427) -> (-5, 20.7927) construction
  line L14 (-5, 20.7927) -> (-5, 22.9427) construction
  circle A1 centre (-5, 22.9427) radius 1.5
  line L15 (-5.7239, 25.0927) -> (-5.7239, 27.0927) construction
  line L16 (-5.7239, 27.0927) -> (-2, 27.125) construction
  line L17 (-2, 27.125) -> (-5.7239, 27.0927)
  line L18 (-5.7239, 25.0927) -> (-5.7239, 27.0927)
  line L19 (-5.7239, 25.0927) -> (-3.7587, 25.0927)
  line L20 (-3.7587, 25.0927) -> (-2.5174, 22.9427)
  line L21 (-2.5174, 22.9427) -> (-3.7587, 20.7927)
  line L22 (-3.7587, 20.7927) -> (-3.7587, 20.5732)
  line L23 (-3.7587, 20.5732) -> (-1.7194, 20.5732)
  line L24 (-1.7194, 20.5732) -> (-1.7194, 27.125)
  line L25 (-2, 27.125) -> (-1.7194, 27.125)
  line L26 (-11.0542, 25.9381) -> (-11.0542, 26.4381)
  point P0 (-2, 2.5)
  point P1 (-2, 2.5)
  point P2 (-4.4826, 22.9427)
  dimension "d205" = 4.3
  dimension "d206" = 3
  dimension "d207" = 2
  dimension "d1051" = 0.5
  constraints: 54 end point, 4 vertical, 3 collinear, 2 centre point, 2 point on circle, 1 coincident, 1 horizontal, 1 midpoint, 1 perpendicular, 1 point on line
  measures "d205" distance of L6.start L6.end
  measures "d206" diameter of A1
  measures "d207" distance of L19.start L15.end
  measures "d1051" distance of L26.start L26.end
extrude "Extrusion13" cut sketch "Sketch15" against normal blind 10 contours A1